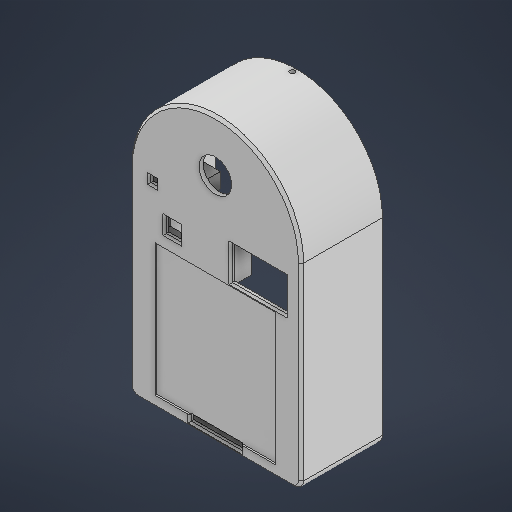
# Autodesk Inventor part: enclouser
Saved by Autodesk Inventor 2026.1 (Build 301233020, 233B)
## iProperties
Created: 2025-12-06
Part Number: enclouser
Material: Generic
Document SubType Name: Modeling
Designer: ASUS
Density: 1 g/cm^3
Appearance: Default
Author: ASUS
Autodesk Inventor part; units mm, degrees
ref_plane "YZ Plane" through (0, 0, 0) normal (1, 0, 0) x (0, 1, 0)
ref_plane "XZ Plane" through (0, 0, 0) normal (0, 1, 0) x (-1, 0, 0)
ref_plane "XY Plane" through (0, 0, 0) normal (0, 0, 1) x (1, 0, 0)
sketch "Sketch1" plane through (0, 0, 0) normal (0, 0, 1) x (1, 0, 0)
  line L0 (50, -70) -> (50, 25)
  line L1 (-50, 25) -> (-50, -70)
  line L2 (0, 0) -> (-38.1854, 57.2781) construction
  arc A0 (50, 25) -> (-50, 25) centre (0, 25) ccw
  line L3 (-45, -90) -> (45, -90)
  line L4 (0, 0) -> (38.1854, 57.2781) construction
  line L5 (50, -70) -> (50, -85)
  line L6 (-50, -70) -> (-50, -85)
  arc A1 (45, -90) -> (50, -85) centre (45, -85) ccw
  arc A2 (-50, -85) -> (-45, -90) centre (-45, -85) ccw
  dimension "d19" = 5
  constraints: 14 end point, 8 point on circle, 6 tangent, 3 centre point, 2 vertical, 1 equal radius, 1 parallel
  measures "d19" radius of A1
extrude "Extrusion1" add sketch "Sketch1" along normal blind 47.5
shell "Shell1" thickness 2.5 removed faces 1 at (-16.6667, -6.6667, 0)
sketch "Sketch2" plane through (0, 25, 45) normal (0, 0, -1) x (-1, 0, 0)
  arc A0 (50, 0) -> (-50, 0) centre (0, 0) ccw projected
  line L0 (25, 0) -> (50, 0) construction
  line L1 (25, 0) -> (50, 0) construction
  line L2 (-25, 0) -> (-50, 0)
  line L3 (-47.5, -110) -> (-47.5, 0) projected
  line L4 (25, 0) -> (50, 0) construction
  line L5 (25, 0) -> (50, 0) construction
  line L6 (47.5, 0) -> (47.5, -112.5)
  line L7 (47.5, -112.5) -> (-47.5, -112.5)
  line L8 (-47.5, -112.5) -> (-47.5, 0)
  line L9 (20.5, -24.5) -> (29.5, -24.5)
  line L10 (29.5, -24.5) -> (29.5, -15.5)
  line L11 (29.5, -15.5) -> (20.5, -15.5)
  line L12 (20.5, -15.5) -> (20.5, -24.5)
  circle A1 centre (25, -20) radius 0.7
  line L13 (20.5, -24.5) -> (29.5, -15.5) construction
  line L14 (29.5, -24.5) -> (20.5, -15.5) construction
  circle A2 centre (36.5, -1.2321) radius 0.9
  line L15 (34.5, 0.7679) -> (38.5, 0.7679)
  line L16 (38.5, -3.2321) -> (34.5, -3.2321)
  line L17 (34.5, 0.7679) -> (38.5, -3.2321) construction
  line L18 (38.5, 0.7679) -> (34.5, -3.2321) construction
  line L19 (34.5, -3.2321) -> (34.5, 0.7679)
  line L20 (29.5, -15.5) -> (29.5, -24.5)
  circle A3 centre (25, -20) radius 0.7
  line L21 (20.5, -15.5) -> (29.5, -15.5)
  line L22 (29.5, -24.5) -> (20.5, -24.5)
  line L23 (20.5, -24.5) -> (20.5, -15.5)
  line L24 (20.5, -15.5) -> (29.5, -24.5) construction
  line L25 (29.5, -15.5) -> (20.5, -24.5) construction
  line L26 (11.5, -30.9599) -> (38.5, -30.9599)
  line L27 (38.5, 9.0401) -> (11.5, 9.0401)
  line L28 (11.5, 9.0401) -> (11.5, -30.9599)
  line L29 (38.5, -30.9599) -> (38.5, 9.0401)
  line L30 (38.5, 0.7679) -> (38.5, -3.2321)
  line L31 (25, -20) -> (25, 0)
  line L32 (-25, 0) -> (-25, -20)
  line L33 (-25, 0) -> (-5, 0) construction
  line L34 (-41, -30) -> (-9, -30)
  line L35 (-9, -30) -> (-9, -10)
  line L36 (-9, -10) -> (-41, -10)
  line L37 (-41, -10) -> (-41, -30)
  line L38 (-41, -30) -> (-9, -10) construction
  line L39 (-9, -30) -> (-41, -10) construction
  line L40 (0, 0) -> (0, 20)
  circle A4 centre (0, 20) radius 9.5
  line L41 (33.5, -108) -> (-35.5, -108)
  line L42 (-35.5, -108) -> (-35.5, -32)
  line L43 (-35.5, -32) -> (33.5, -32)
  line L44 (33.5, -32) -> (33.5, -108)
  line L45 (33.5, -108) -> (-35.5, -32) construction
  line L46 (-35.5, -108) -> (33.5, -32) construction
  line L47 (-15, -112) -> (15, -112)
  line L48 (15, -112) -> (15, -108)
  line L49 (15, -108) -> (-15, -108)
  line L50 (-15, -108) -> (-15, -112)
  line L51 (-15, -112) -> (15, -108) construction
  line L52 (15, -112) -> (-15, -108) construction
  point P0 (0, -25)
  point P1 (-47.5, -95)
  point P2 (25, -20)
  point P3 (-1, -70)
  point P4 (0, -110)
  dimension "d26" = 20
  dimension "d27" = 90
  dimension "d28" = 32
  dimension "d29" = 20
  dimension "d30" = 20
  dimension "d31" = 19
  dimension "d32" = 69
  dimension "d33" = 76
  constraints: 104 end point, 9 midpoint, 9 parallel, 8 horizontal, 6 perpendicular, 4 centre point, 3 vertical, 2 point on line
  measures "d26" distance of L2.start L32.end
  measures "d27" angle of L32 L33
  measures "d28" distance of L36.end L35.end
  measures "d29" distance of L35.end L34.end
  measures "d30" distance of L40.start L40.end
  measures "d31" diameter of A4
  measures "d32" distance of L42.end L43.end
  measures "d33" distance of L41.end L42.end
extrude "Extrusion2" cut sketch "Sketch2" against normal blind 50 contours A1 | L12 L11 L10 L9 | A2 | L15 L29 L16 L19 | L37 L36 L35 L34 | A4 | L48 L47 L50 L41
sketch "Sketch3" plane through (0, 25, 45) normal (0, 0, -1) x (-1, 0, 0)
  line L0 (29.5, -24.5) -> (29.5, -15.5)
  circle A0 centre (25, -20) radius 0.7
  line L1 (20.5, -24.5) -> (29.5, -24.5)
  line L2 (29.5, -15.5) -> (20.5, -15.5)
  line L3 (20.5, -15.5) -> (20.5, -24.5)
  line L4 (20.5, -24.5) -> (29.5, -15.5) construction
  line L5 (29.5, -24.5) -> (20.5, -15.5) construction
  circle A1 centre (36.5, -1.2321) radius 0.9
  line L6 (34.5, 0.7679) -> (38.5, -3.2321) construction
  circle A2 centre (25, -20) radius 0.7
  line L7 (20.5, -15.5) -> (29.5, -15.5)
  line L8 (29.5, -15.5) -> (29.5, -24.5)
  line L9 (29.5, -24.5) -> (20.5, -24.5)
  line L10 (20.5, -24.5) -> (20.5, -15.5)
  line L11 (20.5, -15.5) -> (29.5, -24.5) construction
  line L12 (29.5, -15.5) -> (20.5, -24.5) construction
  line L13 (38.5, -3.2321) -> (34.5, -3.2321)
  line L14 (34.5, -3.2321) -> (34.5, 0.7679)
  line L15 (38.5, 0.7679) -> (38.5, -3.2321)
  line L16 (38.5, 0.7679) -> (34.5, -3.2321) construction
  line L17 (34.5, 0.7679) -> (38.5, 0.7679)
  line L18 (11.5, -30.9599) -> (38.5, -30.9599)
  line L19 (11.5, 9.0401) -> (11.5, -30.9599)
  line L20 (38.5, -30.9599) -> (38.5, 9.0401)
  line L21 (38.5, 9.0401) -> (11.5, 9.0401)
  line L22 (25, -20) -> (25, 0)
  line L23 (-25, 0) -> (-25, -20)
  line L24 (-25, 0) -> (-5, 0) construction
  line L25 (-41, -30) -> (-9, -30)
  line L26 (-9, -30) -> (-9, -10)
  line L27 (-9, -10) -> (-41, -10)
  line L28 (-41, -10) -> (-41, -30)
  line L29 (-41, -30) -> (-9, -10) construction
  line L30 (-9, -30) -> (-41, -10) construction
  line L31 (0, 0) -> (0, 20)
  line L32 (9.5, -32.9599) -> (40.5, -32.9599)
  line L33 (40.5, -32.9599) -> (40.5, 11.0401)
  line L34 (40.5, 11.0401) -> (9.5, 11.0401)
  line L35 (9.5, 11.0401) -> (9.5, -32.9599)
  line L36 (-7, -8) -> (-7, -32)
  line L37 (-43, -32) -> (-43, -8)
  line L38 (-41, -30) -> (-41, -32)
  line L39 (11.25, 9.2901) -> (38.75, 9.2901)
  line L40 (38.75, 9.2901) -> (38.75, -31.2099)
  line L41 (38.75, -31.2099) -> (11.25, -31.2099)
  line L42 (11.25, -31.2099) -> (11.25, 9.2901)
  line L43 (-25, -9.75) -> (-8.75, -9.75)
  line L44 (-8.75, -9.75) -> (-8.75, -30.25)
  line L45 (-8.75, -30.25) -> (-41.25, -30.25)
  line L46 (-41.25, -30.25) -> (-41.25, -9.75)
  line L47 (-41.25, -9.75) -> (-41.25, -8)
  line L48 (-41.25, -30.25) -> (-41.25, -32)
  line L49 (-8.75, -30.25) -> (-8.75, -32)
  line L50 (-8.75, -9.75) -> (-8.75, -8)
  line L51 (-43, -8) -> (-41.25, -8)
  line L52 (-8.75, -8) -> (-7, -8)
  line L53 (-7, -32) -> (-8.75, -32)
  line L54 (-41, -32) -> (-43, -32)
  line L55 (6, -20.0179) -> (44, -20.0179)
  line L56 (44, -20.0179) -> (44, 2.2679)
  line L57 (44, 2.2679) -> (6, 2.2679)
  line L58 (6, 2.2679) -> (6, -20.0179)
  line L59 (6, -20.0179) -> (44, 2.2679) construction
  line L60 (44, -20.0179) -> (6, 2.2679) construction
  point P0 (0, -25)
  point P1 (25, -20)
  point P2 (25, -8.875)
  point P3 (40.5, -20.0179)
  point P4 (38.75, -20.0179)
  point P5 (11.25, -20.0179)
  point P6 (9.5, -20.0179)
  point P7 (9.5, 2.2679)
  point P8 (11.25, 2.2679)
  point P9 (38.75, 2.2679)
  point P10 (40.5, 2.2679)
  dimension "d36" = 20
  dimension "d37" = 90
  dimension "d39" = 20
  dimension "d40" = 20
  dimension "d41" = 2
  dimension "d42" = 0.25
  dimension "d44" = 0.25
  constraints: 122 end point, 13 parallel, 9 perpendicular, 7 midpoint, 5 vertical, 4 point on line, 3 centre point, 3 horizontal, 8 other
  measures "d36" distance of L23.start L23.end
  measures "d37" angle of L23 L24
  measures "d39" distance of L26.end L26.start
  measures "d40" distance of L31.start L31.end
  measures "d41" distance between parallel lines of L19 L35
  measures "d42" distance between parallel lines of L21 L39
  measures "d44" distance between parallel lines of L27 L43
extrude "Extrusion3" add sketch "Sketch3" along normal blind 10 contours L55 L33 L32 L35 L42 L41 L40 | L40 L39 L42 L57 L35 L34 L33 | L50 L52 L36 L53 L49 L44 | L48 L54 L37 L51 L47 L46
chamfer "Chamfer1" distance 1 angle 45 12 edges at (25, 15, 47.5) (41, 5, 47.5) (25, -5, 47.5) (9, 5, 47.5) (-25, 9.5, 47.5) (-20.5, 5, 47.5) (-29.5, 5, 47.5) (-25, 0.5, 47.5) (-36.5, 21.7679, 47.5) (-34.5, 23.7679, 47.5) (-36.5, 25.7679, 47.5) (-38.5, 23.7679, 47.5)
chamfer "Chamfer2" distance 1 angle 45 4 edges at (0, -83, 47.5) (0, -87, 47.5) (-15, -85, 47.5) (15, -85, 47.5)
sketch "Sketch4" plane through (0, 0, 47.5) normal (0, 0, 1) x (1, 0, 0)
  line L0 (15, -83) -> (-15, -83) projected
  line L1 (0, -83) -> (0, -45)
  line L2 (-35, -83.5) -> (35, -83.5)
  line L3 (35, -83.5) -> (35, -6.5)
  line L4 (35, -6.5) -> (-35, -6.5)
  line L5 (-35, -6.5) -> (-35, -83.5)
  line L6 (-35, -83.5) -> (35, -6.5) construction
  line L7 (35, -83.5) -> (-35, -6.5) construction
  point P0 (0, 0)
  dimension "d53" = 38
  dimension "d54" = 70
  dimension "d55" = 77
  constraints: 14 end point, 3 midpoint, 2 parallel, 1 horizontal, 1 perpendicular, 1 vertical
  measures "d53" distance of L1.start L1.end
  measures "d54" distance of L4.end L3.end
  measures "d55" distance of L3.end L2.end
extrude "Extrusion4" cut sketch "Sketch4" against normal blind 1
chamfer "Chamfer3" distance 1.5 angle 45 6 edges at (0, 75, 47.5) (-50, -30, 47.5) (-48.5355, -88.5355, 47.5) (0, -90, 47.5) (48.5355, -88.5355, 47.5) (50, -30, 47.5)
sketch "Sketch5" plane through (-45, -90, 0) normal (0, -1, 0) x (1, 0, 0)
  line L0 (45, 0) -> (45, 5)
  circle A0 centre (45, 2.5) radius 1.45
  dimension "d61" = 5
  dimension "d62" = 2.9
  constraints: 2 end point, 1 centre point, 1 midpoint, 1 vertical
  measures "d61" distance of L0.start L0.end
  measures "d62" diameter of A0
extrude "Extrusion5" cut sketch "Sketch5" against normal through all
body "Solid1"
